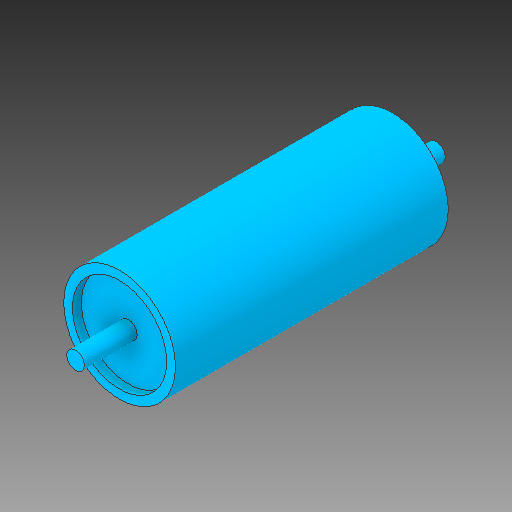
# Autodesk Inventor part: Rodo
Saved by Autodesk Inventor 2019 (Build 230136000, 136)
## iProperties
Created: 2019-02-26
Part Number: Rodo
Material: Generic
Document SubType Name: Modeling
Designer: felix
Density: 1 g/cm^3
Appearance: Default
Mass: 473.105 g
Surface Area: 408.207 cm^2
Volume: 473.105 cm^3
Author: felix
Autodesk Inventor part; units mm, degrees
ref_plane "YZ Plane" through (0, 0, 0) normal (1, 0, 0) x (0, 1, 0)
ref_plane "XZ Plane" through (0, 0, 0) normal (0, 1, 0) x (-1, 0, 0)
ref_plane "XY Plane" through (0, 0, 0) normal (0, 0, 1) x (1, 0, 0)
sketch "Sketch1" plane through (0, 0, 0) normal (0, 0, 1) x (1, 0, 0)
  circle A0 centre (0, 0) radius 31.75
  dimension "d0" = 31.75
  constraints: 1 centre point, 1 coincident
  measures "d0" radius of A0
extrude "Extrusion1" add sketch "Sketch1" along normal mid plane 155
sketch "Sketch2" plane through (0, 0, -77.5) normal (0, 0, -1) x (-1, 0, 0)
  circle A0 centre (0, 0) radius 26.75
  dimension "d3" = 26.75
  constraints: 1 centre point, 1 coincident
  measures "d3" radius of A0
extrude "Extrusion2" cut sketch "Sketch2" against normal blind 5
sketch "Sketch3" plane through (0, 0, 77.5) normal (0, 0, 1) x (1, 0, 0)
  circle A0 centre (0, 0) radius 26.75
  dimension "d6" = 26.75
  constraints: 1 centre point, 1 coincident
  measures "d6" radius of A0
extrude "Extrusion3" cut sketch "Sketch3" against normal blind 5
sketch "Sketch4" plane through (0, 0, -72.5) normal (0, 0, -1) x (-1, 0, 0)
  circle A0 centre (0, 0) radius 5
  dimension "d9" = 5
  constraints: 1 centre point, 1 coincident
  measures "d9" radius of A0
extrude "Extrusion4" add sketch "Sketch4" along normal blind 30
sketch "Sketch5" plane through (0, 0, 72.5) normal (0, 0, 1) x (1, 0, 0)
  circle A0 centre (0, 0) radius 5
  dimension "d12" = 5
  constraints: 1 centre point, 1 coincident
  measures "d12" radius of A0
extrude "Extrusion5" add sketch "Sketch5" along normal blind 30
body "Solid1"
